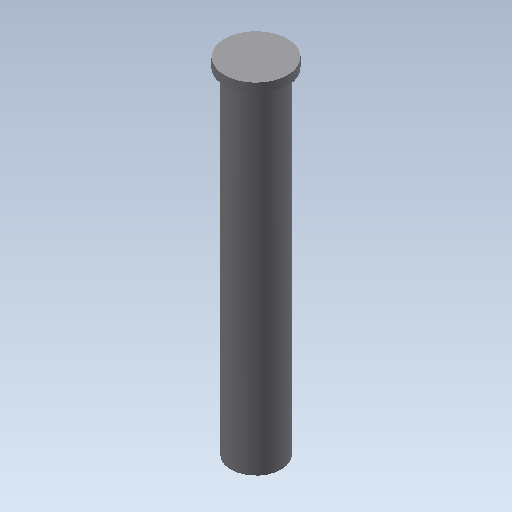
# Autodesk Inventor part: post
Saved by Autodesk Inventor 2020 (Build 240168000, 168)
## iProperties
Created: 2016-10-06
Part Number: post
Material: Genérico
Document SubType Name: Modeling
Designer: i7
Density: 1 g/cm^3
Appearance: Valor por defecto
Author: i7
Autodesk Inventor part; units mm, degrees
ref_plane "YZ Plane" through (0, 0, 0) normal (1, 0, 0) x (0, 1, 0)
ref_plane "XZ Plane" through (0, 0, 0) normal (0, 1, 0) x (-1, 0, 0)
ref_plane "XY Plane" through (0, 0, 0) normal (0, 0, 1) x (1, 0, 0)
sketch "Boceto1" plane through (0, 0, 0) normal (0, 1, 0) x (-1, 0, 0)
  circle A0 centre (0, 0) radius 12.7
  circle A1 centre (0, 0) radius 15.875
  dimension "d0" = 25.4
  dimension "d1" = 31.75
  constraints: 2 centre point, 2 coincident
  measures "d0" diameter of A0
  measures "d1" diameter of A1
extrude "Extrusión1" add sketch "Boceto1" along normal blind 4.7
sketch "Boceto2" plane through (0, 4.7, 0) normal (0, 1, 0) x (1, 0, 0)
  circle A0 centre (0, 0) radius 12.7
  dimension "d4" = 25.4
  constraints: 1 centre point, 1 coincident
  measures "d4" diameter of A0
extrude "Extrusión2" add sketch "Boceto2" against normal blind 173.6
hole "Agujero1" at (0.5939, -168.9, -0.5568) direction (0, 1, 0) diameter 4 depth 8 counterbore diameter 10.2 counterbore depth 0.5
thread "Rosca1" size "M4x0.7" class "6H" standard "ANSI Metric M Profile" full length
